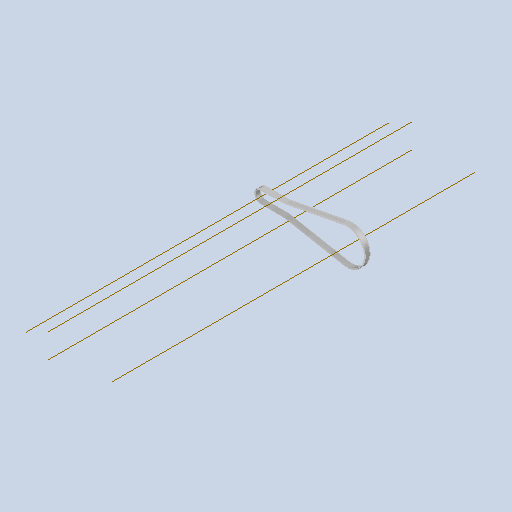
# Autodesk Inventor part: Synchronous Belt
Saved by Autodesk Inventor 2022.2 (Build 262287030, 287C)
## iProperties
CustomPartVersion: 1
Created: 2022-01-10
Part Number: Synchronous Belt
Material: Rubber
Document SubType Name: Modeling
Designer: Jochen
Density: 1 g/cm^3
Appearance: Rubber - Black - Version 1.1
Author: Jochen
Autodesk Inventor part; units mm, degrees
ref_plane "YZ Plane" through (0, 0, 0) normal (1, 0, 0) x (0, 1, 0)
ref_plane "XZ Plane" through (0, 0, 0) normal (0, 1, 0) x (-1, 0, 0)
ref_plane "XY Plane" through (0, 0, 0) normal (0, 0, 1) x (1, 0, 0)
sketch "Sketch Path" plane through (0, 0, 0) normal (0, 0, 1) x (1, 0, 0)
  arc A0 (9.935467, -4.607054) -> (9.935467, -14.155918) centre (9.980951, -9.381486) ccw
  arc A1 (28.387676, -4.431268) -> (29.244844, -4.345803) centre (28.341951, 0.368514) ccw
  arc A2 (76.407011, -23.449739) -> (76.407011, 4.686767) centre (79.101384, -9.381486) ccw
  arc A3 (29.244844, -14.417169) -> (28.387676, -14.331704) centre (28.341951, -19.131486) ccw
  line L0 (28.387676, -14.331704) -> (9.935467, -14.155918)
  line L1 (9.935467, -4.607054) -> (28.387676, -4.431268)
  line L2 (29.244844, -4.345803) -> (76.407011, 4.686767)
  line L3 (76.407011, -23.449739) -> (29.244844, -14.417169)
  constraints: 8 end point, 8 point on circle, 4 centre point
ref_plane "Cross Section Plane" through (9.935467, -14.155918, 0) normal (0.9999546, -0.0095261, 0) x (0, 0, 1)
ref_plane "Work Plane2" through (9.980951, -9.381486, 0) normal (-1, 0, 0) x (0, 0, 1)
ref_plane "Work Plane3" through (79.101384, -9.381486, 0) normal (-0.9828158, -0.184589, 0) x (0, 0, 1)
sketch "Cross Section" plane through (9.935467, -14.155918, 0) normal (0.9999546, -0.0095261, 0) x (0, 0, 1)
  line L0 (-2, 0.3) -> (2, 0.3)
  line L1 (2, 0.3) -> (2, -0.3)
  line L2 (2, -0.3) -> (-2, -0.3)
  line L3 (-2, -0.3) -> (-2, 0.3)
  line L4 (-2, 0) -> (2, 0) construction
  point P0 (0, 0)
  point P1 (0, 0)
  dimension "d0" = 4
  dimension "d4" = 0.3
  dimension "d5" = 0.3
  constraints: 10 end point, 3 midpoint, 2 parallel, 1 coincident, 1 horizontal, 1 perpendicular, 1 other
  measures "d0" distance between parallel lines of L1 L3
  measures "d4" distance between parallel lines of L2 L4
  measures "d5" distance between parallel lines of L4 L0
sweep "Belt" add profiles "Cross Section" path "Sketch Path" path curves L3 A3 L0 A0 L1 A1 L2 A2
equation "\"d0\" = da_B"
equation "\"d4\" = da_a"
equation "\"d5\" = da_a2"
equation "\"da_B\" = 4"
equation "\"da_pb\" = 2.5"
equation "\"da_a\" = 0.3"
equation "\"da_S\" = 1.5"
equation "\"da_Beta\" = 20deg"
equation "\"da_Ht\" = 0.7"
equation "\"da_H\" = 1.3"
equation "\"da_a2\" = 0.3"
body "Solid1"
